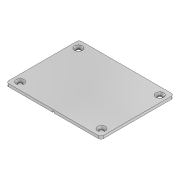
# Autodesk Inventor part: Bed
Saved by Autodesk Inventor 2020 (Build 240168000, 168)
## iProperties
Created: 2020-11-11
Part Number: Bed
Material: Generic
Document SubType Name: Modeling
Designer: ferrerx
Density: 1 g/cm^3
Appearance: Aluminum - Polished
Author: ferrerx
Autodesk Inventor part; units mm, degrees
ref_plane "YZ Plane" through (0, 0, 0) normal (1, 0, 0) x (0, 1, 0)
ref_plane "XZ Plane" through (0, 0, 0) normal (0, 1, 0) x (-1, 0, 0)
ref_plane "XY Plane" through (0, 0, 0) normal (0, 0, 1) x (1, 0, 0)
sketch "Sketch1" plane through (0, 0, 0) normal (0, 1, 0) x (-1, 0, 0)
  line L0 (-35, 27) -> (35, 27)
  line L1 (35, 27) -> (35, -27)
  line L2 (35, -27) -> (-35, -27)
  line L3 (-35, -27) -> (-35, 27)
  line L4 (-35, 27) -> (35, -27) construction
  line L5 (35, 27) -> (-35, -27) construction
  line L6 (30, 21.5) -> (-30, 21.5) construction
  line L7 (-30, 21.5) -> (-30, -21.5) construction
  line L8 (-30, -21.5) -> (30, -21.5) construction
  line L9 (30, -21.5) -> (30, 21.5) construction
  line L10 (30, 21.5) -> (-30, -21.5) construction
  line L11 (-30, 21.5) -> (30, -21.5) construction
  circle A0 centre (30, 21.5) radius 1.5
  circle A1 centre (30, -21.5) radius 1.5
  circle A2 centre (-30, -21.5) radius 1.5
  circle A3 centre (-30, 21.5) radius 1.5
  point P0 (0, 0)
  dimension "d0" = 70
  dimension "d1" = 54
  dimension "d2" = 43
  dimension "d3" = 60
  dimension "d4" = 3
  dimension "d5" = 3
  dimension "d6" = 3
  dimension "d7" = 3
  constraints: 24 end point, 4 centre point, 4 coincident, 4 midpoint, 4 parallel, 2 horizontal, 2 perpendicular
  measures "d0" distance of L1.end L2.end
  measures "d1" distance of L2.end L0.start
  measures "d2" distance of L8.end L6.start
  measures "d3" distance of L7.end L8.end
  measures "d4" diameter of A3
  measures "d5" diameter of A2
  measures "d6" diameter of A1
  measures "d7" diameter of A0
extrude "Extrusion1" add sketch "Sketch1" along normal blind 2
fillet "Fillet1" radius 2 4 edges at (35, 1, 27) (35, 1, -27) (-35, 1, 27) (-35, 1, -27)
sketch "Sketch2" plane through (0, 0, 0) normal (0, -1, 0) x (1, 0, 0)
  circle A0 centre (0, 0) radius 3.5
  dimension "d11" = 7
  constraints: 1 centre point, 1 coincident
  measures "d11" diameter of A0
extrude "Extrusion2" cut sketch "Sketch2" against normal blind 1
sketch "Sketch3" plane through (0, 0, 0) normal (0, -1, 0) x (1, 0, 0)
  line L0 (-33, 27) -> (33, 27) projected
  circle A0 centre (0, 0) radius 3.5 projected
  line L1 (0, 27) -> (0, 0)
  line L2 (0.5, 27) -> (-0.5, 27)
  line L3 (-0.5, 27) -> (-0.5, 0)
  line L4 (-0.5, 0) -> (0.5, 0)
  line L5 (0.5, 0) -> (0.5, 27)
  point P0 (-0.5, 27)
  dimension "d14" = 0.5
  dimension "d15" = 0.5
  constraints: 10 end point, 2 parallel, 1 horizontal, 1 midpoint, 1 perpendicular, 1 point on line, 1 vertical
  measures "d14" distance between parallel lines of L1 L3
  measures "d15" distance between parallel lines of L5 L1
extrude "Extrusion3" cut sketch "Sketch3" against normal blind 1 contours L0 L1 A0 L3 | L0 L5 A0 L1 | A0 L1 L4 L3 | A0 L5 L4 L1
chamfer "Chamfer1" distance 1.4 angle 45 4 edges at (-28.5, 2, -21.5) (-28.5, 2, 21.5) (31.5, 2, 21.5) (31.5, 2, -21.5)
body "Solid1"
